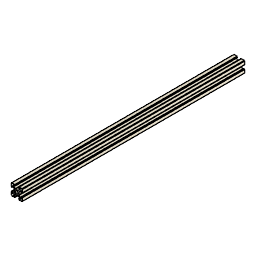
2D Printer Full Assembly (Autodesk Fusion 360 archive; units mm, degrees)
design "2020 400mm T-Slot Extrusion"
Autodesk Fusion 360 part; units mm, degrees
(part 1 of 8)
sketch "profile" plane through (0, 0, 0) normal (0, 1, 0) x (1, 0, 0)
  circle A0 centre (0, 0) radius 2.5
  line L0 (0, -3.9) -> (-2.5, -3.9)
  line L1 (4, -4) -> (-4, 4) construction
  line L2 (-3.9092, -3.9092) -> (4, 4) construction
  line L3 (10, -10) -> (-10, -10) construction
  line L4 (-10, -10) -> (-10, 10) construction
  line L5 (-10, 10) -> (10, 10) construction
  line L6 (10, 10) -> (10, -10) construction
  line L7 (10, -10) -> (-10, 10) construction
  line L8 (-10, -10) -> (10, 10) construction
  line L9 (8, -8) -> (-8, -8) construction
  line L10 (-8, -8) -> (-8, 8) construction
  line L11 (-8, 8) -> (8, 8) construction
  line L12 (8, 8) -> (8, -8) construction
  line L13 (8, -8) -> (-8, 8) construction
  line L14 (-8, -8) -> (8, 8) construction
  line L15 (0, -8) -> (0, -10) construction
  line L16 (0, -9) -> (-3.1, -9) construction
  line L17 (-3.1, -8) -> (-3.1, -9.6)
  line L18 (-1.75, -10) -> (-1.75, -9.6) construction
  line L19 (0, -9.6) -> (-3.5, -9.6) construction
  line L20 (-3.1, -9.6) -> (-3.5, -9.6)
  line L21 (-3.5, -9.6) -> (-3.5, -10)
  line L22 (0, 0) -> (0, -8) construction
  line L23 (-3.5, -10) -> (-10, -10)
  line L24 (-3.9092, -3.9092) -> (-2.5, -3.9) construction
  line L25 (-8, -8) -> (-6.6, -8) construction
  line L26 (-8, -8) -> (-8, -7) construction
  line L27 (-2.5, -3.9) -> (-6.6, -8)
  line L28 (-6.6, -8) -> (-3.1, -8)
  line L29 (0, -2.5) -> (0, -3.9) construction
  line L30 (-3.9, 0) -> (-3.9, -2.5)
  line L31 (-3.9, -2.5) -> (-8, -6.6)
  line L32 (-8, -6.6) -> (-8, -3.1)
  line L33 (-8, -3.1) -> (-9.6, -3.1)
  line L34 (-9.6, -3.1) -> (-9.6, -3.5)
  line L35 (-9.6, -3.5) -> (-10, -3.5)
  line L36 (-10, -3.5) -> (-10, -10)
  line L37 (0, 0) -> (10, 0) construction
  line L38 (3.9, 0) -> (3.9, -2.5)
  line L39 (3.9, -2.5) -> (8, -6.6)
  line L40 (8, -6.6) -> (8, -3.1)
  line L41 (8, -3.1) -> (9.6, -3.1)
  line L42 (9.6, -3.1) -> (9.6, -3.5)
  line L43 (9.6, -3.5) -> (10, -3.5)
  line L44 (10, -3.5) -> (10, -10)
  line L45 (0, -3.9) -> (2.5, -3.9)
  line L46 (6.6, -8) -> (3.1, -8)
  line L47 (3.1, -8) -> (3.1, -9.6)
  line L48 (3.1, -9.6) -> (3.5, -9.6)
  line L49 (3.5, -9.6) -> (3.5, -10)
  line L50 (3.5, -10) -> (10, -10)
  line L51 (2.5, -3.9) -> (6.6, -8)
  line L52 (-3.9, 0) -> (-3.9, 2.5)
  line L53 (-3.9, 2.5) -> (-8, 6.6)
  line L54 (-8, 6.6) -> (-8, 3.1)
  line L55 (-8, 3.1) -> (-9.6, 3.1)
  line L56 (-9.6, 3.1) -> (-9.6, 3.5)
  line L57 (-9.6, 3.5) -> (-10, 3.5)
  line L58 (-10, 3.5) -> (-10, 10)
  line L59 (0, 3.9) -> (-2.5, 3.9)
  line L60 (-6.6, 8) -> (-3.1, 8)
  line L61 (-3.1, 8) -> (-3.1, 9.6)
  line L62 (-3.1, 9.6) -> (-3.5, 9.6)
  line L63 (-3.5, 9.6) -> (-3.5, 10)
  line L64 (-3.5, 10) -> (-10, 10)
  line L65 (-2.5, 3.9) -> (-6.6, 8)
  line L66 (0, 3.9) -> (2.5, 3.9)
  line L67 (6.6, 8) -> (3.1, 8)
  line L68 (3.1, 8) -> (3.1, 9.6)
  line L69 (3.1, 9.6) -> (3.5, 9.6)
  line L70 (3.5, 9.6) -> (3.5, 10)
  line L71 (3.5, 10) -> (10, 10)
  line L72 (2.5, 3.9) -> (6.6, 8)
  line L73 (3.9, 0) -> (3.9, 2.5)
  line L74 (8, 6.6) -> (8, 3.1)
  line L75 (8, 3.1) -> (9.6, 3.1)
  line L76 (9.6, 3.1) -> (9.6, 3.5)
  line L77 (9.6, 3.5) -> (10, 3.5)
  line L78 (10, 3.5) -> (10, 10)
  line L79 (3.9, 2.5) -> (8, 6.6)
  dimension "d3" = 5
  dimension "d7" = 8
  dimension "d8" = 8
  dimension "d9" = 20
  dimension "d10" = 20
  dimension "d11" = 16
  dimension "d12" = 16
  dimension "d13" = 3.1
  dimension "d14" = 0.4
  dimension "d15" = 3.5
  dimension "d20" = 2.5
  dimension "d21" = 1.4
  constraint coincident A0.centre L22.start
  constraint horizontal L0
  constraint coincident L1 A0.centre
  constraint coincident L2 A0.centre
  constraint horizontal L3
  constraint perpendicular L3 L4
  constraint parallel L3 L5
  constraint parallel L4 L6
  constraint coincident L7 A0.centre
  constraint coincident L8 A0.centre
  constraint horizontal L9
  constraint perpendicular L9 L10
  constraint parallel L9 L11
  constraint parallel L10 L12
  constraint coincident L13 A0.centre
  constraint coincident L14 A0.centre
  constraint midpoint L9 L15.start
  constraint midpoint L3 L15.end
  constraint midpoint L15 L16.start
  constraint perpendicular L15 L16
  constraint coincident L9 L17.start
  constraint perpendicular L3 L17
  constraint coincident L16.end L17
  constraint vertical L18
  constraint coincident L3 L18.start
  constraint coincident L15 L19.start
  constraint perpendicular L15 L19
  constraint coincident L18.end L19
  constraint coincident L19 L17.end
  constraint coincident L3 L21.end
  constraint perpendicular L3 L21
  constraint midpoint L18.end L19
  constraint coincident L9 L25.end
  constraint coincident L10 L26.end
  constraint parallel L14 L27
  constraint coincident L22 L0.start
  constraint coincident L22 L29.start
  constraint coincident A0 L29.start
  constraint parallel L22 L29
  constraint coincident L0.start L29.end
  constraint symmetric L3.end L8 L4.start
  constraint symmetric L8 L17.start L32.end
  constraint symmetric L8 L19.end L34.end
  constraint symmetric L8 L17.end L33.end
  constraint symmetric L8 L21.end L35.end
  constraint symmetric L8 L0.end L30.end
  constraint symmetric L8 L25.end L31.end
  constraint symmetric L8 L0.start L30.start
  constraint midpoint L6 L37.end
  constraint symmetric L3.end L22 L3.start
  constraint symmetric L17.start L22 L46.end
  constraint symmetric L19.end L22 L48.end
  constraint symmetric L17.end L22 L47.end
  constraint symmetric L21.end L22 L49.end
  constraint symmetric L22 L0.end L45.end
  constraint symmetric L22 L25.end L46.start
  constraint symmetric L22 L0.start L29.end
  constraint symmetric L22 L30.start L38.start
  constraint symmetric L22 L30.end L38.end
  constraint symmetric L22 L31.end L39.end
  constraint symmetric L22 L32.end L40.end
  constraint symmetric L22 L33.end L41.end
  constraint symmetric L22 L34.end L42.end
  constraint symmetric L22 L35.end L43.end
  constraint symmetric L22 L3.end L3.start
  constraint symmetric L3.end L37 L4.end
  constraint symmetric L17.start L37 L60.end
  constraint symmetric L19.end L37 L62.end
  constraint symmetric L17.end L37 L61.end
  constraint symmetric L21.end L37 L63.end
  constraint symmetric L0.end L37 L59.end
  constraint symmetric L25.end L37 L60.start
  constraint symmetric L0.start L37 L59.start
  constraint symmetric L30.start L37 L52.start
  constraint symmetric L30.end L37 L52.end
  constraint symmetric L31.end L37 L53.end
  constraint symmetric L32.end L37 L54.end
  constraint symmetric L33.end L37 L55.end
  constraint symmetric L34.end L37 L56.end
  constraint symmetric L35.end L37 L57.end
  constraint symmetric L37 L38.start L73.start
  constraint symmetric L37 L38.end L73.end
  constraint symmetric L37 L39.end L74.start
  constraint symmetric L37 L40.end L74.end
  constraint symmetric L37 L41.end L75.end
  constraint symmetric L37 L42.end L76.end
  constraint symmetric L37 L43.end L77.end
  constraint symmetric L37 L3.start L5.end
  constraint symmetric L37 L0.start L59.start
  constraint symmetric L37 L45.end L66.end
  constraint symmetric L37 L46.start L67.start
  constraint symmetric L37 L46.end L67.end
  constraint symmetric L37 L47.end L68.end
  constraint symmetric L37 L48.end L69.end
  constraint symmetric L37 L49.end L70.end
  measures "d3" diameter of A0
  measures "d7" distance of L1.end L2.end
  measures "d8" distance of L1.start L2.end
  measures "d9" distance of L4.end L5.end
  measures "d10" distance of L3.end L4.end
  measures "d11" distance of L10.end L11.end
  measures "d12" distance of L9.end L10.end
  measures "d13" distance of L16.start L16.end
  measures "d14" distance of L18.start L18.end
  measures "d15" distance of L19.start L19.end
  measures "d20" distance of L0.end L0.start
  measures "d21" distance of L29.start L0.start
extrude "Extrude3" add sketch "profile" along normal blind 400
fillet "Fillet1" radius 0.6 4 edges at (-10, 200, 10) (10, 200, 10) (10, 200, -10) (-10, 200, -10)
fillet "Fillet1" radius 0.2 8 edges at (3.1, 200, 8) (8, 200, 3.1) (8, 200, -3.1) (3.1, 200, -8) (-3.1, 200, 8) (-8, 200, 3.1) (-3.1, 200, -8) (-8, 200, -3.1)
fillet "Fillet1" radius 0.2 8 edges at (-8, 200, 6.6) (-6.6, 200, 8) (6.6, 200, 8) (8, 200, 6.6) (8, 200, -6.6) (6.6, 200, -8) (-6.6, 200, -8) (-8, 200, -6.6)
fillet "Fillet1" radius 0.4 8 edges at (-2.5, 200, 3.9) (2.5, 200, 3.9) (3.9, 200, 2.5) (3.9, 200, -2.5) (2.5, 200, -3.9) (-2.5, 200, -3.9) (-3.9, 200, -2.5) (-3.9, 200, 2.5)
equation "d13 = ( 6.2 / 2 ) * 1 mm"
equation "d15 = 7 mm / 2"

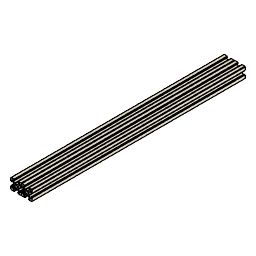
design "2040 400mm T-Slot Extrusion"
Autodesk Fusion 360 part; units mm, degrees
sketch "profile" plane through (0, 0, 0) normal (0, 1, 0) x (1, 0, 0)
  circle A0 centre (0, 0) radius 2.5
  line L0 (0, -3.9) -> (-2.5, -3.9)
  line L1 (4, -4) -> (-4, 4) construction
  line L2 (-3.9092, -3.9092) -> (4, 4) construction
  line L3 (10, -10) -> (-10, -10) construction
  line L4 (-10, -10) -> (-10, 10) construction
  line L5 (-10, 10) -> (10, 10) construction
  line L6 (10, 10) -> (10, -10) construction
  line L7 (10, -10) -> (-10, 10) construction
  line L8 (-10, -10) -> (10, 10) construction
  line L9 (8, -8) -> (-8, -8) construction
  line L10 (-8, -8) -> (-8, 8) construction
  line L11 (-8, 8) -> (8, 8) construction
  line L12 (8, 8) -> (8, -8) construction
  line L13 (8, -8) -> (-8, 8) construction
  line L14 (-8, -8) -> (8, 8) construction
  line L15 (0, -8) -> (0, -10) construction
  line L16 (0, -9) -> (-3.1, -9) construction
  line L17 (-3.1, -8) -> (-3.1, -9.6)
  line L18 (-1.75, -10) -> (-1.75, -9.6) construction
  line L19 (0, -9.6) -> (-3.5, -9.6) construction
  line L20 (-3.1, -9.6) -> (-3.5, -9.6)
  line L21 (-3.5, -9.6) -> (-3.5, -10)
  line L22 (0, 0) -> (0, -8) construction
  line L23 (-3.5, -10) -> (-10, -10)
  line L24 (-3.9092, -3.9092) -> (-2.5, -3.9) construction
  line L25 (-8, -8) -> (-6.6, -8) construction
  line L26 (-8, -8) -> (-8, -7) construction
  line L27 (-2.5, -3.9) -> (-6.6, -8)
  line L28 (-6.6, -8) -> (-3.1, -8)
  line L29 (0, -2.5) -> (0, -3.9) construction
  line L30 (-3.9, 0) -> (-3.9, -2.5)
  line L31 (-3.9, -2.5) -> (-8, -6.6)
  line L32 (-8, -6.6) -> (-8, -3.1)
  line L33 (-8, -3.1) -> (-9.6, -3.1)
  line L34 (-9.6, -3.1) -> (-9.6, -3.5)
  line L35 (-9.6, -3.5) -> (-10, -3.5)
  line L36 (-10, -3.5) -> (-10, -10)
  line L37 (0, 0) -> (10, 0) construction
  line L38 (3.9, 0) -> (3.9, -2.5)
  line L39 (3.9, -2.5) -> (8, -6.6)
  line L40 (8, -6.6) -> (8, -3.1)
  line L41 (8, -3.1) -> (9.6, -3.1)
  line L42 (9.6, -3.1) -> (9.6, -3.5)
  line L43 (9.6, -3.5) -> (10, -3.5)
  line L44 (10, -3.5) -> (10, -10)
  line L45 (0, -3.9) -> (2.5, -3.9)
  line L46 (6.6, -8) -> (3.1, -8)
  line L47 (3.1, -8) -> (3.1, -9.6)
  line L48 (3.1, -9.6) -> (3.5, -9.6)
  line L49 (3.5, -9.6) -> (3.5, -10)
  line L50 (3.5, -10) -> (10, -10)
  line L51 (2.5, -3.9) -> (6.6, -8)
  line L52 (-3.9, 0) -> (-3.9, 2.5)
  line L53 (-3.9, 2.5) -> (-8, 6.6)
  line L54 (-8, 6.6) -> (-8, 3.1)
  line L55 (-8, 3.1) -> (-9.6, 3.1)
  line L56 (-9.6, 3.1) -> (-9.6, 3.5)
  line L57 (-9.6, 3.5) -> (-10, 3.5)
  line L58 (-10, 3.5) -> (-10, 10)
  line L59 (0, 3.9) -> (-2.5, 3.9)
  line L60 (-6.6, 8) -> (-3.1, 8)
  line L61 (-3.1, 8) -> (-3.1, 9.6)
  line L62 (-3.1, 9.6) -> (-3.5, 9.6)
  line L63 (-3.5, 9.6) -> (-3.5, 10)
  line L64 (-3.5, 10) -> (-10, 10)
  line L65 (-2.5, 3.9) -> (-6.6, 8)
  line L66 (0, 3.9) -> (2.5, 3.9)
  line L67 (6.6, 8) -> (3.1, 8)
  line L68 (3.1, 8) -> (3.1, 9.6)
  line L69 (3.1, 9.6) -> (3.5, 9.6)
  line L70 (3.5, 9.6) -> (3.5, 10)
  line L71 (3.5, 10) -> (10, 10)
  line L72 (2.5, 3.9) -> (6.6, 8)
  line L73 (3.9, 0) -> (3.9, 2.5)
  line L74 (8, 6.6) -> (8, 3.1)
  line L75 (8, 3.1) -> (9.6, 3.1)
  line L76 (9.6, 3.1) -> (9.6, 3.5)
  line L77 (9.6, 3.5) -> (10, 3.5)
  line L78 (10, 3.5) -> (10, 10)
  line L79 (3.9, 2.5) -> (8, 6.6)
  dimension "d3" = 5
  dimension "d7" = 8
  dimension "d8" = 8
  dimension "d9" = 20
  dimension "d10" = 20
  dimension "d11" = 16
  dimension "d12" = 16
  dimension "d13" = 3.1
  dimension "d14" = 0.4
  dimension "d15" = 3.5
  dimension "d20" = 2.5
  dimension "d21" = 1.4
  constraint coincident A0.centre L22.start
  constraint horizontal L0
  constraint coincident L1 A0.centre
  constraint coincident L2 A0.centre
  constraint horizontal L3
  constraint perpendicular L3 L4
  constraint parallel L3 L5
  constraint parallel L4 L6
  constraint coincident L7 A0.centre
  constraint coincident L8 A0.centre
  constraint horizontal L9
  constraint perpendicular L9 L10
  constraint parallel L9 L11
  constraint parallel L10 L12
  constraint coincident L13 A0.centre
  constraint coincident L14 A0.centre
  constraint midpoint L9 L15.start
  constraint midpoint L3 L15.end
  constraint midpoint L15 L16.start
  constraint perpendicular L15 L16
  constraint coincident L9 L17.start
  constraint perpendicular L3 L17
  constraint coincident L16.end L17
  constraint vertical L18
  constraint coincident L3 L18.start
  constraint coincident L15 L19.start
  constraint perpendicular L15 L19
  constraint coincident L18.end L19
  constraint coincident L19 L17.end
  constraint coincident L3 L21.end
  constraint perpendicular L3 L21
  constraint midpoint L18.end L19
  constraint coincident L9 L25.end
  constraint coincident L10 L26.end
  constraint parallel L14 L27
  constraint coincident L22 L0.start
  constraint coincident L22 L29.start
  constraint coincident A0 L29.start
  constraint parallel L22 L29
  constraint coincident L0.start L29.end
  constraint symmetric L3.end L8 L4.start
  constraint symmetric L8 L17.start L32.end
  constraint symmetric L8 L19.end L34.end
  constraint symmetric L8 L17.end L33.end
  constraint symmetric L8 L21.end L35.end
  constraint symmetric L8 L0.end L30.end
  constraint symmetric L8 L25.end L31.end
  constraint symmetric L8 L0.start L30.start
  constraint midpoint L6 L37.end
  constraint symmetric L3.end L22 L3.start
  constraint symmetric L17.start L22 L46.end
  constraint symmetric L19.end L22 L48.end
  constraint symmetric L17.end L22 L47.end
  constraint symmetric L21.end L22 L49.end
  constraint symmetric L22 L0.end L45.end
  constraint symmetric L22 L25.end L46.start
  constraint symmetric L22 L0.start L29.end
  constraint symmetric L22 L30.start L38.start
  constraint symmetric L22 L30.end L38.end
  constraint symmetric L22 L31.end L39.end
  constraint symmetric L22 L32.end L40.end
  constraint symmetric L22 L33.end L41.end
  constraint symmetric L22 L34.end L42.end
  constraint symmetric L22 L35.end L43.end
  constraint symmetric L22 L3.end L3.start
  constraint symmetric L3.end L37 L4.end
  constraint symmetric L17.start L37 L60.end
  constraint symmetric L19.end L37 L62.end
  constraint symmetric L17.end L37 L61.end
  constraint symmetric L21.end L37 L63.end
  constraint symmetric L0.end L37 L59.end
  constraint symmetric L25.end L37 L60.start
  constraint symmetric L0.start L37 L59.start
  constraint symmetric L30.start L37 L52.start
  constraint symmetric L30.end L37 L52.end
  constraint symmetric L31.end L37 L53.end
  constraint symmetric L32.end L37 L54.end
  constraint symmetric L33.end L37 L55.end
  constraint symmetric L34.end L37 L56.end
  constraint symmetric L35.end L37 L57.end
  constraint symmetric L37 L38.start L73.start
  constraint symmetric L37 L38.end L73.end
  constraint symmetric L37 L39.end L74.start
  constraint symmetric L37 L40.end L74.end
  constraint symmetric L37 L41.end L75.end
  constraint symmetric L37 L42.end L76.end
  constraint symmetric L37 L43.end L77.end
  constraint symmetric L37 L3.start L5.end
  constraint symmetric L37 L0.start L59.start
  constraint symmetric L37 L45.end L66.end
  constraint symmetric L37 L46.start L67.start
  constraint symmetric L37 L46.end L67.end
  constraint symmetric L37 L47.end L68.end
  constraint symmetric L37 L48.end L69.end
  constraint symmetric L37 L49.end L70.end
  measures "d3" diameter of A0
  measures "d7" distance of L1.end L2.end
  measures "d8" distance of L1.start L2.end
  measures "d9" distance of L4.end L5.end
  measures "d10" distance of L3.end L4.end
  measures "d11" distance of L10.end L11.end
  measures "d12" distance of L9.end L10.end
  measures "d13" distance of L16.start L16.end
  measures "d14" distance of L18.start L18.end
  measures "d15" distance of L19.start L19.end
  measures "d20" distance of L0.end L0.start
  measures "d21" distance of L29.start L0.start
extrude "Extrude3" add sketch "profile" along normal blind 400 makes body 1
fillet "Fillet1" radius 0.6 4 edges at (-10, 200, 10) (10, 200, 10) (10, 200, -10) (-10, 200, -10) on bodies 1
fillet "Fillet1" radius 0.2 8 edges at (3.1, 200, 8) (8, 200, 3.1) (8, 200, -3.1) (3.1, 200, -8) (-3.1, 200, 8) (-8, 200, 3.1) (-3.1, 200, -8) (-8, 200, -3.1) on bodies 1
fillet "Fillet1" radius 0.2 8 edges at (-8, 200, 6.6) (-6.6, 200, 8) (6.6, 200, 8) (8, 200, 6.6) (8, 200, -6.6) (6.6, 200, -8) (-6.6, 200, -8) (-8, 200, -6.6) on bodies 1
fillet "Fillet1" radius 0.4 8 edges at (-2.5, 200, 3.9) (2.5, 200, 3.9) (3.9, 200, 2.5) (3.9, 200, -2.5) (2.5, 200, -3.9) (-2.5, 200, -3.9) (-3.9, 200, -2.5) (-3.9, 200, 2.5) on bodies 1
copy_body "CopyPasteBodies1" bodies 1 makes body 2
move_body "Move1" bodies 2 to x (1, 0, 0) y (0, 1, 0) z (0, 0, 1) at (-20, 0, 0)
equation "d13 = ( 6.2 / 2 ) * 1 mm"
equation "d15 = 7 mm / 2"

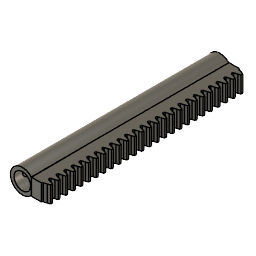
design "Rack Pen Holder"
description: Rack; Circular Pitch: 4.12283 mm; Num Teeth: 26; Pressure Angle: 20 deg; Backlash: 0.12 mm;
Autodesk Fusion 360 part; units mm, degrees
sketch "Sketch1" plane through (0, 0, 0) normal (0, 0, 1) x (1, 0, 0) in component "Rack; Circular Pitch: 4.12283 mm; Num Teeth: 26; Pressure Angle: 20 deg; Backlash: 0.12 mm;"
  line L0 (-1.7283, -1.4496) -> (0, -0.9707)
  line L1 (0, -0.9707) -> (1.3123, -0.4931)
  line L2 (-1.7283, 1.4496) -> (0, 0.9707)
  line L3 (0, 0.9707) -> (1.3123, 0.4931)
  line L4 (1.3123, 0.4931) -> (1.3123, -0.4931)
  line L5 (-2.0948, 1.9315) -> (-2.0948, 2.0614)
  line L6 (-2.0948, -1.9315) -> (-2.0948, -2.0614)
  arc A0 (-2.0948, 1.9315) -> (-1.7283, 1.4496) centre (-1.5948, 1.9315) ccw
  arc A1 (-1.7283, -1.4496) -> (-2.0948, -1.9315) centre (-1.5948, -1.9315) ccw
  line L7 (-1.7283, 2.6732) -> (0, 3.1521)
  line L8 (0, 3.1521) -> (1.3123, 3.6298)
  line L9 (-1.7283, 5.5724) -> (0, 5.0935)
  line L10 (0, 5.0935) -> (1.3123, 4.6159)
  line L11 (1.3123, 4.6159) -> (1.3123, 3.6298)
  line L12 (-2.0948, 6.0543) -> (-2.0948, 6.1842)
  line L13 (-2.0948, 2.1914) -> (-2.0948, 2.0614)
  arc A2 (-2.0948, 6.0543) -> (-1.7283, 5.5724) centre (-1.5948, 6.0543) ccw
  arc A3 (-1.7283, 2.6732) -> (-2.0948, 2.1914) centre (-1.5948, 2.1914) ccw
  line L14 (-1.7283, 6.796) -> (0, 7.275)
  line L15 (0, 7.275) -> (1.3123, 7.7526)
  line L16 (-1.7283, 9.6953) -> (0, 9.2164)
  line L17 (0, 9.2164) -> (1.3123, 8.7387)
  line L18 (1.3123, 8.7387) -> (1.3123, 7.7526)
  line L19 (-2.0948, 10.1771) -> (-2.0948, 10.3071)
  line L20 (-2.0948, 6.3142) -> (-2.0948, 6.1842)
  arc A4 (-2.0948, 10.1771) -> (-1.7283, 9.6953) centre (-1.5948, 10.1771) ccw
  arc A5 (-1.7283, 6.796) -> (-2.0948, 6.3142) centre (-1.5948, 6.3142) ccw
  line L21 (-1.7283, 10.9189) -> (0, 11.3978)
  line L22 (0, 11.3978) -> (1.3123, 11.8754)
  line L23 (-1.7283, 13.8181) -> (0, 13.3392)
  line L24 (0, 13.3392) -> (1.3123, 12.8615)
  line L25 (1.3123, 12.8615) -> (1.3123, 11.8754)
  line L26 (-2.0948, 14.3) -> (-2.0948, 14.4299)
  line L27 (-2.0948, 10.437) -> (-2.0948, 10.3071)
  arc A6 (-2.0948, 14.3) -> (-1.7283, 13.8181) centre (-1.5948, 14.3) ccw
  arc A7 (-1.7283, 10.9189) -> (-2.0948, 10.437) centre (-1.5948, 10.437) ccw
  line L28 (-1.7283, 15.0417) -> (0, 15.5206)
  line L29 (0, 15.5206) -> (1.3123, 15.9983)
  line L30 (-1.7283, 17.9409) -> (0, 17.462)
  line L31 (0, 17.462) -> (1.3123, 16.9844)
  line L32 (1.3123, 16.9844) -> (1.3123, 15.9983)
  line L33 (-2.0948, 18.4228) -> (-2.0948, 18.5527)
  line L34 (-2.0948, 14.5599) -> (-2.0948, 14.4299)
  arc A8 (-2.0948, 18.4228) -> (-1.7283, 17.9409) centre (-1.5948, 18.4228) ccw
  arc A9 (-1.7283, 15.0417) -> (-2.0948, 14.5599) centre (-1.5948, 14.5599) ccw
  line L35 (-1.7283, 19.1645) -> (0, 19.6434)
  line L36 (0, 19.6434) -> (1.3123, 20.1211)
  line L37 (-1.7283, 22.0638) -> (0, 21.5849)
  line L38 (0, 21.5849) -> (1.3123, 21.1072)
  line L39 (1.3123, 21.1072) -> (1.3123, 20.1211)
  line L40 (-2.0948, 22.5456) -> (-2.0948, 22.6756)
  line L41 (-2.0948, 18.6827) -> (-2.0948, 18.5527)
  arc A10 (-2.0948, 22.5456) -> (-1.7283, 22.0638) centre (-1.5948, 22.5456) ccw
  arc A11 (-1.7283, 19.1645) -> (-2.0948, 18.6827) centre (-1.5948, 18.6827) ccw
  line L42 (-1.7283, 23.2874) -> (0, 23.7663)
  line L43 (0, 23.7663) -> (1.3123, 24.2439)
  line L44 (-1.7283, 26.1866) -> (0, 25.7077)
  line L45 (0, 25.7077) -> (1.3123, 25.23)
  line L46 (1.3123, 25.23) -> (1.3123, 24.2439)
  line L47 (-2.0948, 26.6684) -> (-2.0948, 26.7984)
  line L48 (-2.0948, 22.8055) -> (-2.0948, 22.6756)
  arc A12 (-2.0948, 26.6684) -> (-1.7283, 26.1866) centre (-1.5948, 26.6684) ccw
  arc A13 (-1.7283, 23.2874) -> (-2.0948, 22.8055) centre (-1.5948, 22.8055) ccw
  line L49 (-1.7283, 27.4102) -> (0, 27.8891)
  line L50 (0, 27.8891) -> (1.3123, 28.3668)
  line L51 (-1.7283, 30.3094) -> (0, 29.8305)
  line L52 (0, 29.8305) -> (1.3123, 29.3529)
  line L53 (1.3123, 29.3529) -> (1.3123, 28.3668)
  line L54 (-2.0948, 30.7913) -> (-2.0948, 30.9212)
  line L55 (-2.0948, 26.9283) -> (-2.0948, 26.7984)
  arc A14 (-2.0948, 30.7913) -> (-1.7283, 30.3094) centre (-1.5948, 30.7913) ccw
  arc A15 (-1.7283, 27.4102) -> (-2.0948, 26.9283) centre (-1.5948, 26.9283) ccw
  line L56 (-1.7283, 31.533) -> (0, 32.0119)
  line L57 (0, 32.0119) -> (1.3123, 32.4896)
  line L58 (-1.7283, 34.4323) -> (0, 33.9533)
  line L59 (0, 33.9533) -> (1.3123, 33.4757)
  line L60 (1.3123, 33.4757) -> (1.3123, 32.4896)
  line L61 (-2.0948, 34.9141) -> (-2.0948, 35.0441)
  line L62 (-2.0948, 31.0512) -> (-2.0948, 30.9212)
  arc A16 (-2.0948, 34.9141) -> (-1.7283, 34.4323) centre (-1.5948, 34.9141) ccw
  arc A17 (-1.7283, 31.533) -> (-2.0948, 31.0512) centre (-1.5948, 31.0512) ccw
  line L63 (-1.7283, 35.6559) -> (0, 36.1348)
  line L64 (0, 36.1348) -> (1.3123, 36.6124)
  line L65 (-1.7283, 38.5551) -> (0, 38.0762)
  line L66 (0, 38.0762) -> (1.3123, 37.5985)
  line L67 (1.3123, 37.5985) -> (1.3123, 36.6124)
  line L68 (-2.0948, 39.0369) -> (-2.0948, 39.1669)
  line L69 (-2.0948, 35.174) -> (-2.0948, 35.0441)
  arc A18 (-2.0948, 39.0369) -> (-1.7283, 38.5551) centre (-1.5948, 39.0369) ccw
  arc A19 (-1.7283, 35.6559) -> (-2.0948, 35.174) centre (-1.5948, 35.174) ccw
  line L70 (-1.7283, 39.7787) -> (0, 40.2576)
  line L71 (0, 40.2576) -> (1.3123, 40.7352)
  line L72 (-1.7283, 42.6779) -> (0, 42.199)
  line L73 (0, 42.199) -> (1.3123, 41.7214)
  line L74 (1.3123, 41.7214) -> (1.3123, 40.7352)
  line L75 (-2.0948, 43.1598) -> (-2.0948, 43.2897)
  line L76 (-2.0948, 39.2968) -> (-2.0948, 39.1669)
  arc A20 (-2.0948, 43.1598) -> (-1.7283, 42.6779) centre (-1.5948, 43.1598) ccw
  arc A21 (-1.7283, 39.7787) -> (-2.0948, 39.2968) centre (-1.5948, 39.2968) ccw
  line L77 (-1.7283, 43.9015) -> (0, 44.3804)
  line L78 (0, 44.3804) -> (1.3123, 44.8581)
  line L79 (-1.7283, 46.8007) -> (0, 46.3218)
  line L80 (0, 46.3218) -> (1.3123, 45.8442)
  line L81 (1.3123, 45.8442) -> (1.3123, 44.8581)
  line L82 (-2.0948, 47.2826) -> (-2.0948, 47.4125)
  line L83 (-2.0948, 43.4197) -> (-2.0948, 43.2897)
  arc A22 (-2.0948, 47.2826) -> (-1.7283, 46.8007) centre (-1.5948, 47.2826) ccw
  arc A23 (-1.7283, 43.9015) -> (-2.0948, 43.4197) centre (-1.5948, 43.4197) ccw
  line L84 (-1.7283, 48.0243) -> (0, 48.5033)
  line L85 (0, 48.5033) -> (1.3123, 48.9809)
  line L86 (-1.7283, 50.9236) -> (0, 50.4447)
  line L87 (0, 50.4447) -> (1.3123, 49.967)
  line L88 (1.3123, 49.967) -> (1.3123, 48.9809)
  line L89 (-2.0948, 51.4054) -> (-2.0948, 51.5354)
  line L90 (-2.0948, 47.5425) -> (-2.0948, 47.4125)
  arc A24 (-2.0948, 51.4054) -> (-1.7283, 50.9236) centre (-1.5948, 51.4054) ccw
  arc A25 (-1.7283, 48.0243) -> (-2.0948, 47.5425) centre (-1.5948, 47.5425) ccw
  line L91 (-1.7283, 52.1472) -> (0, 52.6261)
  line L92 (0, 52.6261) -> (1.3123, 53.1037)
  line L93 (-1.7283, 55.0464) -> (0, 54.5675)
  line L94 (0, 54.5675) -> (1.3123, 54.0898)
  line L95 (1.3123, 54.0898) -> (1.3123, 53.1037)
  line L96 (-2.0948, 55.5283) -> (-2.0948, 55.6582)
  line L97 (-2.0948, 51.6653) -> (-2.0948, 51.5354)
  arc A26 (-2.0948, 55.5283) -> (-1.7283, 55.0464) centre (-1.5948, 55.5283) ccw
  arc A27 (-1.7283, 52.1472) -> (-2.0948, 51.6653) centre (-1.5948, 51.6653) ccw
  line L98 (-1.7283, 56.27) -> (0, 56.7489)
  line L99 (0, 56.7489) -> (1.3123, 57.2266)
  line L100 (-1.7283, 59.1692) -> (0, 58.6903)
  line L101 (0, 58.6903) -> (1.3123, 58.2127)
  line L102 (1.3123, 58.2127) -> (1.3123, 57.2266)
  line L103 (-2.0948, 59.6511) -> (-2.0948, 59.781)
  line L104 (-2.0948, 55.7882) -> (-2.0948, 55.6582)
  arc A28 (-2.0948, 59.6511) -> (-1.7283, 59.1692) centre (-1.5948, 59.6511) ccw
  arc A29 (-1.7283, 56.27) -> (-2.0948, 55.7882) centre (-1.5948, 55.7882) ccw
  line L105 (-1.7283, 60.3928) -> (0, 60.8717)
  line L106 (0, 60.8717) -> (1.3123, 61.3494)
  line L107 (-1.7283, 63.2921) -> (0, 62.8132)
  line L108 (0, 62.8132) -> (1.3123, 62.3355)
  line L109 (1.3123, 62.3355) -> (1.3123, 61.3494)
  line L110 (-2.0948, 63.7739) -> (-2.0948, 63.9039)
  line L111 (-2.0948, 59.911) -> (-2.0948, 59.781)
  arc A30 (-2.0948, 63.7739) -> (-1.7283, 63.2921) centre (-1.5948, 63.7739) ccw
  arc A31 (-1.7283, 60.3928) -> (-2.0948, 59.911) centre (-1.5948, 59.911) ccw
  line L112 (-1.7283, 64.5157) -> (0, 64.9946)
  line L113 (0, 64.9946) -> (1.3123, 65.4722)
  line L114 (-1.7283, 67.4149) -> (0, 66.936)
  line L115 (0, 66.936) -> (1.3123, 66.4583)
  line L116 (1.3123, 66.4583) -> (1.3123, 65.4722)
  line L117 (-2.0948, 67.8967) -> (-2.0948, 68.0267)
  line L118 (-2.0948, 64.0338) -> (-2.0948, 63.9039)
  arc A32 (-2.0948, 67.8967) -> (-1.7283, 67.4149) centre (-1.5948, 67.8967) ccw
  arc A33 (-1.7283, 64.5157) -> (-2.0948, 64.0338) centre (-1.5948, 64.0338) ccw
  line L119 (-1.7283, 68.6385) -> (0, 69.1174)
  line L120 (0, 69.1174) -> (1.3123, 69.5951)
  line L121 (-1.7283, 71.5377) -> (0, 71.0588)
  line L122 (0, 71.0588) -> (1.3123, 70.5812)
  line L123 (1.3123, 70.5812) -> (1.3123, 69.5951)
  line L124 (-2.0948, 72.0196) -> (-2.0948, 72.1495)
  line L125 (-2.0948, 68.1566) -> (-2.0948, 68.0267)
  arc A34 (-2.0948, 72.0196) -> (-1.7283, 71.5377) centre (-1.5948, 72.0196) ccw
  arc A35 (-1.7283, 68.6385) -> (-2.0948, 68.1566) centre (-1.5948, 68.1566) ccw
  line L126 (-1.7283, 72.7613) -> (0, 73.2402)
  line L127 (0, 73.2402) -> (1.3123, 73.7179)
  line L128 (-1.7283, 75.6606) -> (0, 75.1816)
  line L129 (0, 75.1816) -> (1.3123, 74.704)
  line L130 (1.3123, 74.704) -> (1.3123, 73.7179)
  line L131 (-2.0948, 76.1424) -> (-2.0948, 76.2724)
  line L132 (-2.0948, 72.2795) -> (-2.0948, 72.1495)
  arc A36 (-2.0948, 76.1424) -> (-1.7283, 75.6606) centre (-1.5948, 76.1424) ccw
  arc A37 (-1.7283, 72.7613) -> (-2.0948, 72.2795) centre (-1.5948, 72.2795) ccw
  line L133 (-1.7283, 76.8842) -> (0, 77.3631)
  line L134 (0, 77.3631) -> (1.3123, 77.8407)
  line L135 (-1.7283, 79.7834) -> (0, 79.3045)
  line L136 (0, 79.3045) -> (1.3123, 78.8268)
  line L137 (1.3123, 78.8268) -> (1.3123, 77.8407)
  line L138 (-2.0948, 80.2652) -> (-2.0948, 80.3952)
  line L139 (-2.0948, 76.4023) -> (-2.0948, 76.2724)
  arc A38 (-2.0948, 80.2652) -> (-1.7283, 79.7834) centre (-1.5948, 80.2652) ccw
  arc A39 (-1.7283, 76.8842) -> (-2.0948, 76.4023) centre (-1.5948, 76.4023) ccw
  line L140 (-1.7283, 81.007) -> (0, 81.4859)
  line L141 (0, 81.4859) -> (1.3123, 81.9635)
  line L142 (-1.7283, 83.9062) -> (0, 83.4273)
  line L143 (0, 83.4273) -> (1.3123, 82.9497)
  line L144 (1.3123, 82.9497) -> (1.3123, 81.9635)
  line L145 (-2.0948, 84.3881) -> (-2.0948, 84.518)
  line L146 (-2.0948, 80.5251) -> (-2.0948, 80.3952)
  arc A40 (-2.0948, 84.3881) -> (-1.7283, 83.9062) centre (-1.5948, 84.3881) ccw
  arc A41 (-1.7283, 81.007) -> (-2.0948, 80.5251) centre (-1.5948, 80.5251) ccw
  line L147 (-1.7283, 85.1298) -> (0, 85.6087)
  line L148 (0, 85.6087) -> (1.3123, 86.0864)
  line L149 (-1.7283, 88.029) -> (0, 87.5501)
  line L150 (0, 87.5501) -> (1.3123, 87.0725)
  line L151 (1.3123, 87.0725) -> (1.3123, 86.0864)
  line L152 (-2.0948, 88.5109) -> (-2.0948, 88.6408)
  line L153 (-2.0948, 84.648) -> (-2.0948, 84.518)
  arc A42 (-2.0948, 88.5109) -> (-1.7283, 88.029) centre (-1.5948, 88.5109) ccw
  arc A43 (-1.7283, 85.1298) -> (-2.0948, 84.648) centre (-1.5948, 84.648) ccw
  line L154 (-1.7283, 89.2526) -> (0, 89.7316)
  line L155 (0, 89.7316) -> (1.3123, 90.2092)
  line L156 (-1.7283, 92.1519) -> (0, 91.673)
  line L157 (0, 91.673) -> (1.3123, 91.1953)
  line L158 (1.3123, 91.1953) -> (1.3123, 90.2092)
  line L159 (-2.0948, 92.6337) -> (-2.0948, 92.7637)
  line L160 (-2.0948, 88.7708) -> (-2.0948, 88.6408)
  arc A44 (-2.0948, 92.6337) -> (-1.7283, 92.1519) centre (-1.5948, 92.6337) ccw
  arc A45 (-1.7283, 89.2526) -> (-2.0948, 88.7708) centre (-1.5948, 88.7708) ccw
  line L161 (-1.7283, 93.3755) -> (0, 93.8544)
  line L162 (0, 93.8544) -> (1.3123, 94.332)
  line L163 (-1.7283, 96.2747) -> (0, 95.7958)
  line L164 (0, 95.7958) -> (1.3123, 95.3181)
  line L165 (1.3123, 95.3181) -> (1.3123, 94.332)
  line L166 (-2.0948, 96.7566) -> (-2.0948, 96.8865)
  line L167 (-2.0948, 92.8936) -> (-2.0948, 92.7637)
  arc A46 (-2.0948, 96.7566) -> (-1.7283, 96.2747) centre (-1.5948, 96.7566) ccw
  arc A47 (-1.7283, 93.3755) -> (-2.0948, 92.8936) centre (-1.5948, 92.8936) ccw
  line L168 (-1.7283, 97.4983) -> (0, 97.9772)
  line L169 (0, 97.9772) -> (1.3123, 98.4549)
  line L170 (-1.7283, 100.3975) -> (0, 99.9186)
  line L171 (0, 99.9186) -> (1.3123, 99.441)
  line L172 (1.3123, 99.441) -> (1.3123, 98.4549)
  line L173 (-2.0948, 100.8794) -> (-2.0948, 101.0093)
  line L174 (-2.0948, 97.0165) -> (-2.0948, 96.8865)
  arc A48 (-2.0948, 100.8794) -> (-1.7283, 100.3975) centre (-1.5948, 100.8794) ccw
  arc A49 (-1.7283, 97.4983) -> (-2.0948, 97.0165) centre (-1.5948, 97.0165) ccw
  line L175 (-1.7283, 101.6211) -> (0, 102.1)
  line L176 (0, 102.1) -> (1.3123, 102.5777)
  line L177 (-1.7283, 104.5204) -> (0, 104.0415)
  line L178 (0, 104.0415) -> (1.3123, 103.5638)
  line L179 (1.3123, 103.5638) -> (1.3123, 102.5777)
  line L180 (-2.0948, 105.0022) -> (-2.0948, 105.1322)
  line L181 (-2.0948, 101.1393) -> (-2.0948, 101.0093)
  arc A50 (-2.0948, 105.0022) -> (-1.7283, 104.5204) centre (-1.5948, 105.0022) ccw
  arc A51 (-1.7283, 101.6211) -> (-2.0948, 101.1393) centre (-1.5948, 101.1393) ccw
  line L182 (-1.7283, 105.744) -> (0, 106.2229)
  line L183 (0, 106.2229) -> (1.3123, 106.7005)
  line L184 (-1.7283, 108.6432) -> (0, 108.1643)
  line L185 (0, 108.1643) -> (1.3123, 107.6866)
  line L186 (1.3123, 107.6866) -> (1.3123, 106.7005)
  line L187 (-2.0948, 109.125) -> (-2.0948, 109.255)
  line L188 (-2.0948, 105.2621) -> (-2.0948, 105.1322)
  arc A52 (-2.0948, 109.125) -> (-1.7283, 108.6432) centre (-1.5948, 109.125) ccw
  arc A53 (-1.7283, 105.744) -> (-2.0948, 105.2621) centre (-1.5948, 105.2621) ccw
  line L189 (-2.0948, -2.0614) -> (-7.5948, -2.0614)
  line L190 (-7.5948, -2.0614) -> (-8.0948, 105.1322)
  line L191 (-8.0948, 105.1322) -> (-2.0948, 105.1322)
  constraint tangent L2 A0
  constraint tangent L5 A0
  constraint tangent L0 A1
  constraint tangent L6 A1
  constraint tangent L9 A2
  constraint tangent L12 A2
  constraint tangent L7 A3
  constraint tangent L13 A3
  constraint tangent L16 A4
  constraint tangent L19 A4
  constraint tangent L14 A5
  constraint tangent L20 A5
  constraint tangent L23 A6
  constraint tangent L26 A6
  constraint tangent L21 A7
  constraint tangent L27 A7
  constraint tangent L30 A8
  constraint tangent L33 A8
  constraint tangent L28 A9
  constraint tangent L34 A9
  constraint tangent L37 A10
  constraint tangent L40 A10
  constraint tangent L35 A11
  constraint tangent L41 A11
  constraint tangent L44 A12
  constraint tangent L47 A12
  constraint tangent L42 A13
  constraint tangent L48 A13
  constraint tangent L51 A14
  constraint tangent L54 A14
  constraint tangent L49 A15
  constraint tangent L55 A15
  constraint tangent L58 A16
  constraint tangent L61 A16
  constraint tangent L56 A17
  constraint tangent L62 A17
  constraint tangent L65 A18
  constraint tangent L68 A18
  constraint tangent L63 A19
  constraint tangent L69 A19
  constraint tangent L72 A20
  constraint tangent L75 A20
  constraint tangent L70 A21
  constraint tangent L76 A21
  constraint tangent L79 A22
  constraint tangent L82 A22
  constraint tangent L77 A23
  constraint tangent L83 A23
  constraint tangent L86 A24
  constraint tangent L89 A24
  constraint tangent L84 A25
  constraint tangent L90 A25
  constraint tangent L93 A26
  constraint tangent L96 A26
  constraint tangent L91 A27
  constraint tangent L97 A27
  constraint tangent L100 A28
  constraint tangent L103 A28
  constraint tangent L98 A29
  constraint tangent L104 A29
  constraint tangent L107 A30
  constraint tangent L110 A30
  constraint tangent L105 A31
  constraint tangent L111 A31
  constraint tangent L114 A32
  constraint tangent L117 A32
  constraint tangent L112 A33
  constraint tangent L118 A33
  constraint tangent L121 A34
  constraint tangent L124 A34
  constraint tangent L119 A35
  constraint tangent L125 A35
  constraint tangent L128 A36
  constraint tangent L131 A36
  constraint tangent L126 A37
  constraint tangent L132 A37
  constraint tangent L135 A38
  constraint tangent L138 A38
  constraint tangent L133 A39
  constraint tangent L139 A39
  constraint tangent L142 A40
  constraint tangent L145 A40
  constraint tangent L140 A41
  constraint tangent L146 A41
  constraint tangent L149 A42
  constraint tangent L152 A42
  constraint tangent L147 A43
  constraint tangent L153 A43
  constraint tangent L156 A44
  constraint tangent L159 A44
  constraint tangent L154 A45
  constraint tangent L160 A45
  constraint tangent L163 A46
  constraint tangent L166 A46
  constraint tangent L161 A47
  constraint tangent L167 A47
  constraint tangent L170 A48
  constraint tangent L173 A48
  constraint tangent L168 A49
  constraint tangent L174 A49
  constraint tangent L177 A50
  constraint tangent L180 A50
  constraint tangent L175 A51
  constraint tangent L181 A51
  constraint tangent L184 A52
  constraint tangent L187 A52
  constraint tangent L182 A53
  constraint tangent L188 A53
extrude "Extrude1" add sketch "Sketch1" along normal blind 4.5 and the other way blind 4.5 makes body 1 in component "Rack; Circular Pitch: 4.12283 mm; Num Teeth: 26; Pressure Angle: 20 deg; Backlash: 0.12 mm;"
sketch "Sketch2" plane through (0, 0, 0) normal (0, 0, 1) x (1, 0, 0) in component "Rack; Circular Pitch: 4.12283 mm; Num Teeth: 26; Pressure Angle: 20 deg; Backlash: 0.12 mm;"
  line L0 (0, 0) -> (0, 103.0708) construction